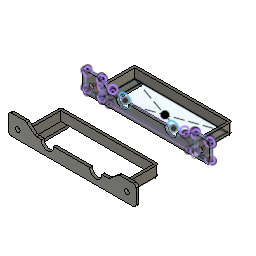
Slate bracket (Autodesk Fusion 360 design; units mm, degrees)
Autodesk Fusion 360 part; units mm, degrees
note: some values were not read from the file. Set by a fixed rule: which sketch regions a step uses.
sketch "Sketch1" plane through (0, 0, 0) normal (0, 0, 1) x (1, 0, 0)
  line L0 (34.5, 12) -> (-34.5, 12)
  line L1 (-34.5, 12) -> (-34.5, -12)
  line L2 (-34.5, -12) -> (34.5, -12)
  line L3 (34.5, -12) -> (34.5, 12)
  line L4 (34.5, 12) -> (-34.5, -12) construction
  line L5 (-34.5, 12) -> (34.5, -12) construction
  line L6 (34.5, 12) -> (29.5, 12)
  line L7 (29.5, 12) -> (29.5, -12)
  line L8 (29.5, -12) -> (34.5, -12)
  line L9 (34.5, -12) -> (34.5, 12)
  line L10 (-34.5, 12) -> (-29.5, 12)
  line L11 (-29.5, 12) -> (-29.5, -12)
  line L12 (-29.5, -12) -> (-34.5, -12)
  line L13 (-34.5, -12) -> (-34.5, 12)
  line L14 (-34.5, -12) -> (-47.5, -12)
  line L15 (-47.5, -12) -> (-47.5, -14)
  line L16 (-47.5, -14) -> (-34.5, -14)
  line L17 (-34.5, -14) -> (-34.5, -12)
  line L18 (34.5, -12) -> (47.5, -12)
  line L19 (47.5, -12) -> (47.5, -14)
  line L20 (47.5, -14) -> (34.5, -14)
  line L21 (34.5, -14) -> (34.5, -12)
  dimension "d1" = 69
  dimension "d2" = 24
  dimension "d9" = 5
  dimension "d10" = 5
  dimension "d14" = 13
  dimension "d15" = 2
  dimension "d16" = 13
  dimension "d17" = 2
  constraint horizontal L0
  constraint perpendicular L0 L1
  constraint parallel L0 L2
  constraint parallel L1 L3
  constraint coincident L4 origin
  constraint coincident L5 origin
  constraint horizontal L6
  constraint vertical L7
  constraint horizontal L8
  constraint vertical L9
  constraint coincident L2 L7.end
  constraint horizontal L10
  constraint vertical L11
  constraint horizontal L12
  constraint vertical L13
  constraint coincident L2 L11.end
  constraint horizontal L14
  constraint vertical L15
  constraint horizontal L16
  constraint vertical L17
  constraint horizontal L18
  constraint vertical L19
  constraint horizontal L20
  constraint vertical L21
  measures "d1" distance of L1.end L2.end
  measures "d2" distance of L0.end L1.end
  measures "d9" distance of L0.start L6.end
  measures "d10" distance of L0.end L10.end
  measures "d14" distance of L1.end L14.end
  measures "d15" distance of L1.end L16.end
  measures "d16" distance of L2.end L18.end
  measures "d17" distance of L2.end L20.end
extrude "Extrude1" add sketch "Sketch1" along normal blind 7 contours L0 L2 L3 L6 L7 L8 L9 | L0 L2 L7 L11 | L0 L1 L2 L10 L11 L12 L13 makes body 1
shell "Shell1" thickness 2 outward yes removed faces 1 at (-9.8333, 4, 7) on bodies 1
extrude "Extrude2" add sketch "Sketch1" along normal blind 13 contours L18 L19 L20 L21 | L14 L15 L16 L17 bodies 1
extrude "Extrude3" cut sketch "Sketch1" against normal through all contours L0 L2 L7 L11 bodies 1
chamfer "Chamfer1" distance 7 distance2 6 2 edges at (-34.5, -13, 7) (34.5, -13, 7) measured on face at (-11.5, -12.6667, 7) measured on face at (-11.5, -12.6667, 7) on bodies 1
extrude "Extrude4" add sketch "Sketch1" against normal blind 2 contours L18 L19 L20 L21 | L14 L15 L16 L17 bodies 1
fillet "Fillet1" radius 2 13 edges at (27.5, -13, 7) (34.5, -13, 13) (47.5, -13, 13) (-27.5, -13, 7) (-34.5, -13, 13) (-47.5, -13, 13) (-36.5, 14, 2.5) (36.5, 14, 2.5) (0, 14, -2) (36.5, 1, -2) (-36.5, 1, -2) (-47.5, -13, -2) (47.5, -13, -2) on bodies 1
sketch "Sketch2" plane through (0, -12, 0) normal (0, 1, 0) x (-1, 0, 0)
  line L0 (-36.5, 7) -> (-34.5, 7)
  line L1 (-34.5, 7) -> (-34.5, 0)
  line L2 (-34.5, 0) -> (-29.5, 0)
  line L3 (-29.5, 0) -> (-29.5, -2)
  line L4 (-45.5, -2) -> (-34.5, -2)
  line L5 (29.5, -2) -> (29.5, 0)
  line L6 (29.5, 0) -> (34.5, 0)
  line L7 (34.5, 0) -> (34.5, 7)
  line L8 (-46.9142, 11.9142) -> (-34.5, 11.9142)
  line L9 (-34.5, 11.9142) -> (-34.5, -2.5)
  line L10 (-34.5, -2.5) -> (-46.9142, -2.5)
  line L11 (-46.9142, -2.5) -> (-46.9142, 11.9142)
  line L12 (46.9142, 12.4142) -> (34.5, 12.4142)
  line L13 (34.5, 12.4142) -> (34.5, -2)
  line L14 (34.5, -2) -> (46.9142, -2)
  line L15 (46.9142, -2) -> (46.9142, 12.4142)
  line L16 (-46.9142, 11.9142) -> (-34.5, -2.5) construction
  line L17 (-46.9142, -2.5) -> (-34.5, 11.9142) construction
  line L18 (34.5, 12.4142) -> (46.9142, -2) construction
  line L19 (46.9142, 12.4142) -> (34.5, -2) construction
  line L20 (34.5, 0) -> (-34.5, 0)
  line L21 (34.5, 6.5) -> (-34.5, 6.5) construction
  circle A0 centre (17.5, 6.5) radius 4.5
  circle A1 centre (-18.5, 6.5) radius 4.5
  arc A2 (-47.5, 0) -> (-45.5, -2) centre (-45.5, 0) ccw
  arc A3 (-36.5, 0) -> (-34.5, -2) centre (-34.5, 0) ccw
  line L22 (-36.5, 0) -> (-36.5, 7)
  line L23 (-29.5, -2) -> (29.5, -2)
  line L24 (34.5, 7) -> (36.5, 7)
  line L25 (36.5, 7) -> (36.5, 0)
  arc A4 (34.5, -2) -> (36.5, 0) centre (34.5, 0) ccw
  line L26 (34.5, -2) -> (45.5, -2)
  arc A5 (45.5, -2) -> (47.5, 0) centre (45.5, 0) ccw
  line L27 (47.5, 0) -> (47.5, 11)
  arc A6 (47.5, 11) -> (45.5, 13) centre (45.5, 11) ccw
  line L28 (45.5, 13) -> (35.2398, 13)
  arc A7 (35.2398, 13) -> (33.9383, 12.5185) centre (35.2398, 11) ccw
  line L29 (33.9383, 12.5185) -> (28.0617, 7.4815)
  arc A8 (26.7602, 7) -> (28.0617, 7.4815) centre (26.7602, 9) ccw
  line L30 (26.7602, 7) -> (-26.7602, 7)
  arc A9 (-28.0617, 7.4815) -> (-26.7602, 7) centre (-26.7602, 9) ccw
  line L31 (-28.0617, 7.4815) -> (-33.9383, 12.5185)
  arc A10 (-33.9383, 12.5185) -> (-35.2398, 13) centre (-35.2398, 11) ccw
  line L32 (-35.2398, 13) -> (-45.5, 13)
  arc A11 (-45.5, 13) -> (-47.5, 11) centre (-45.5, 11) ccw
  line L33 (-47.5, 11) -> (-47.5, 0)
  point P0 (-40.7071, 4.7071)
  point P1 (40.7071, 5.2071)
  point P2 (34.5, 7)
  dimension "d37" = 6.5
  dimension "d38" = 9
  dimension "d39" = 9
  dimension "d40" = 16
  dimension "d44" = 36
  constraint horizontal L8
  constraint vertical L9
  constraint horizontal L10
  constraint vertical L11
  constraint horizontal L12
  constraint vertical L13
  constraint horizontal L14
  constraint vertical L15
  constraint midpoint L16 P0
  constraint midpoint L18 P1
  constraint horizontal L21
  constraint coincident L9 L21.end
  constraint coincident L13 L21.start
  constraint coincident L21 A0.centre
  constraint coincident L21 A1.centre
  measures "d37" distance of L20 L21
  measures "d38" diameter of A0
  measures "d39" diameter of A1
  measures "d40" distance of L9 A1.centre
  measures "d44" distance of A0.centre A1.centre
hole "Hole1" at (40.7071, -12, 4.7071) at (-40.7071, -12, 5.2071) direction (0, -1, 0) diameter 3.5 end through all bodies 1
fillet "Fillet2" radius 1 6 edges at (35.5, -12, 7) (36.5, -12, 3.5) (35.9142, -12, -1.4142) (-35.9142, -12, -1.4142) (-36.5, -12, 3.5) (-35.5, -12, 7) on bodies 1
sketch "Sketch3" plane through (0, 0, -2) normal (0, 0, -1) x (1, 0, 0)
  line L0 (45.5, 12) -> (45.5, 14)
  line L1 (45.5, 14) -> (-45.5, 14)
  line L2 (-45.5, 14) -> (-45.5, 12)
  line L3 (-45.5, 12) -> (-36.7361, 12)
  spline S0 degree 3 poles (-34.5, 11) (-34.8965, 11.2804) (-35.3754, 11.6124) (-36.0968, 11.9123) (-36.4405, 12) (-36.7361, 12) knots 0 0 0 0 0.145689 0.145689 0.234365 0.234365 0.234365 0.234365
  line L4 (-34.5, 11) -> (-34.5, -12)
  line L5 (-34.5, -12) -> (-29.5, -12)
  line L6 (-29.5, -12) -> (-29.5, 12)
  line L7 (-29.5, 12) -> (29.5, 12)
  line L8 (29.5, 12) -> (29.5, -12)
  line L9 (29.5, -12) -> (34.5, -12)
  line L10 (34.5, -12) -> (34.5, 11)
  spline S1 degree 3 poles (36.7361, 12) (36.4405, 12) (36.0968, 11.9123) (35.3754, 11.6124) (34.8965, 11.2804) (34.5, 11) knots 0.566831 0.566831 0.566831 0.566831 0.655508 0.655508 0.801197 0.801197 0.801197 0.801197
  line L11 (36.7361, 12) -> (45.5, 12)
  line L12 (-29.5, -12) -> (29.5, -12)
  line L13 (29.5, -12) -> (29.5, -14)
  line L14 (29.5, -14) -> (-29.5, -14)
  line L15 (-29.5, -14) -> (-29.5, -12)
  line L16 (34.5, -12) -> (-34.5, -12)
  line L17 (-34.5, -14) -> (-34.5, -12)
  line L18 (-29.5, -12) -> (-29.5, 12)
  line L19 (29.5, -12) -> (29.5, 12)
  constraint horizontal L12
  constraint vertical L13
  constraint horizontal L14
  constraint vertical L15
  constraint coincident L5.end L16
  constraint collinear L15 L18
  constraint collinear L13 L19
extrude "Extrude5" cut sketch "Sketch3" against normal blind 2 contours L12 L13 L14 L15 L16 bodies 1
extrude "Extrude6" cut sketch "Sketch2" against normal blind 2 contours A1 L30 | A1 L30 | A0 L30 | A0 L30 bodies 1
mirror "Mirror1" about plane through (0, 0, 0) normal (0, 0, 1) of bodies 1 makes body 2
move_body "Move1" bodies 2 to x (1, 0, 0) y (0, 1, 0) z (0, 0, 1) at (0, 0, 35)
move_body "Move2" bodies 2 to x (-1, 0, 0) y (0, 1, 0) z (0, 0, -1) at (0, 0, 0)
move_body "Move3" bodies 2 to x (1, 0, 0) y (0, 1, 0) z (0, 0, 1) at (0, -55, 35)
named bodies: "Slate bracket left", "Slate bracket right"
